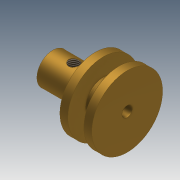
# Autodesk Inventor part: slider-2
Saved by Autodesk Inventor 2017 (Build 210142000, 142)
## iProperties
Created: 2018-09-03
Part Number: slider-2
Material: Brass, Soft Yellow
Document SubType Name: Modeling
Designer: Luiz Gustavo
Density: 8.47 g/cm^3
Appearance: Brass - Satin
Author: Luiz Gustavo
Autodesk Inventor part; units mm, degrees
ref_plane "YZ Plane" through (0, 0, 0) normal (1, 0, 0) x (0, 1, 0)
ref_plane "XZ Plane" through (0, 0, 0) normal (0, 1, 0) x (-1, 0, 0)
ref_plane "XY Plane" through (0, 0, 0) normal (0, 0, 1) x (1, 0, 0)
sketch "Sketch1" plane through (0, 0, 0) normal (0, 1, 0) x (-1, 0, 0)
  line L0 (-10.5, 0) -> (10.5, 0)
  line L1 (-10.5, 1.5) -> (-10.5, 10)
  line L2 (-10.5, 10) -> (-8.25, 10)
  line L3 (-8.25, 10) -> (-8.25, 5)
  line L4 (-8.25, 5) -> (-3.75, 5)
  line L5 (-3.75, 5) -> (-3.75, 10)
  line L6 (-3.75, 10) -> (-1.5, 10)
  line L7 (-1.5, 10) -> (-1.5, 4.5)
  line L8 (-1.5, 4.5) -> (10.5, 4.5)
  line L9 (10.5, 4.5) -> (10.5, 1.5)
  line L10 (10.5, 1.5) -> (-10.5, 1.5)
  line L11 (-10.5, 1.5) -> (-10.5, 0) construction
  line L12 (10.5, 1.5) -> (10.5, 0) construction
  line L13 (-8.25, 10) -> (-3.75, 10) construction
  line L14 (-6, 5) -> (-6, 1.5) construction
  line L15 (4.5, 4) -> (4.5, 1.5) construction
  point P0 (0, 0)
  point P1 (0, 0)
  dimension "d0" = 21
  dimension "d1" = 3
  dimension "d2" = 20
  dimension "d3" = 10
  dimension "d4" = 9
  dimension "d5" = 4.5
  dimension "d6" = 16.5
  dimension "d7" = 12
  dimension "d10" = 6
  constraints: 32 end point, 8 perpendicular, 4 point on line, 3 vertical, 2 collinear, 2 midpoint, 1 coincident, 1 horizontal
  measures "d0" distance of L0.start L0.end
  measures "d1" diameter of L10 L0
  measures "d2" diameter of L2 L0
  measures "d3" diameter of L4 L0
  measures "d4" diameter of L8 L0
  measures "d5" distance between parallel lines of L3 L5
  measures "d6" distance between parallel lines of L14 L9
  measures "d7" distance between parallel lines of L7 L9
  measures "d10" distance between parallel lines of L15 L9
revolve "Revolution1" add sketch "Sketch1" angle 360 about axis through (10.5, 0, 0) along (-1, 0, 0)
sketch "Sketch2" plane through (0, 0, 0) normal (0, 0, 1) x (1, 0, 0)
  circle A0 centre (-4.5, 0) radius 1.5
  line L0 (-3.5, 4) -> (-3.5, -4) projected
  line L1 (-5.5, 4) -> (-5.5, -4) projected
  line L2 (-3.5, 0) -> (-5.5, 0) construction
  line L3 (1.5, 4.5) -> (1.5, -4.5) construction
  point P0 (0, 0)
  dimension "d12" = 3
  constraints: 2 end point, 2 midpoint, 1 centre point, 2 other
  measures "d12" diameter of A0
extrude "Extrusion1" cut sketch "Sketch2" along normal through all both and the other way through all
thread "Thread1" size "M3x0.5" class "6H" standard "ANSI Metric M Profile" full length
equation "\"d13\" = d12"
body "Solid1"
